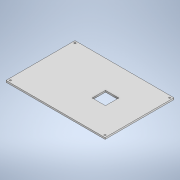
# Autodesk Inventor part: remoteswitchlid
Saved by Autodesk Inventor 2021 (Build 250183000, 183)
## iProperties
Created: 2021-10-23
Part Number: remoteswitchlid
Material: Generic
Document SubType Name: Modeling
Designer: eddys
Density: 1 g/cm^3
Appearance: Default
Author: eddys
Autodesk Inventor part; units mm, degrees
ref_plane "YZ Plane" through (0, 0, 0) normal (1, 0, 0) x (0, 1, 0)
ref_plane "XZ Plane" through (0, 0, 0) normal (0, 1, 0) x (-1, 0, 0)
ref_plane "XY Plane" through (0, 0, 0) normal (0, 0, 1) x (1, 0, 0)
sketch "Sketch1" plane through (0, 0, 0) normal (0, 1, 0) x (-1, 0, 0)
  line L0 (45.25, 31.5) -> (-45.25, 31.5)
  line L1 (-45.25, 31.5) -> (-45.25, -31.5)
  line L2 (-45.25, -31.5) -> (45.25, -31.5)
  line L3 (45.25, -31.5) -> (45.25, 31.5)
  line L4 (45.25, 31.5) -> (-45.25, -31.5) construction
  line L5 (-45.25, 31.5) -> (45.25, -31.5) construction
  point P0 (0, 0)
  dimension "d0" = 63
  dimension "d1" = 90.5
  constraints: 12 end point, 2 midpoint, 2 parallel, 1 horizontal, 1 perpendicular
  measures "d0" distance of L2.end L0.start
  measures "d1" distance of L1.end L2.end
extrude "Extrusion1" add sketch "Sketch1" along normal blind 1.5
sketch "Sketch2" plane through (0, 1.5, 0) normal (0, 1, 0) x (1, 0, 0)
  circle A0 centre (-43.25, -29.5) radius 0.75
  line L0 (-45.25, 31.5) -> (-45.25, -31.5) projected
  line L1 (-45.25, -31.5) -> (45.25, -31.5) projected
  circle A1 centre (-43.25, 29.5) radius 0.75
  line L2 (45.25, 31.5) -> (-45.25, 31.5) projected
  circle A2 centre (43.25, -29.5) radius 0.75
  line L3 (45.25, -31.5) -> (45.25, 31.5) projected
  circle A3 centre (43.25, 29.5) radius 0.75
  point P0 (0, 0)
  dimension "d4" = 2
  dimension "d5" = 2
  dimension "d6" = 1.5
  dimension "d7" = 2
  dimension "d8" = 2
  dimension "d9" = 1.5
  dimension "d10" = 2
  dimension "d11" = 2
  dimension "d12" = 1.5
  dimension "d13" = 1.5
  dimension "d14" = 2
  dimension "d15" = 2
  constraints: 4 centre point
  measures "d4" distance from line of L0 A0.centre
  measures "d5" distance from line of L1 A0.centre
  measures "d6" diameter of A0
  measures "d7" distance from line of L0 A1.centre
  measures "d8" distance from line of L2 A1.centre
  measures "d9" diameter of A1
  measures "d10" distance from line of L1 A2.centre
  measures "d11" distance from line of L3 A2.centre
  measures "d12" diameter of A2
  measures "d13" diameter of A3
  measures "d14" distance from line of L2 A3.centre
  measures "d15" distance from line of L3 A3.centre
extrude "Extrusion2" cut sketch "Sketch2" against normal blind 1.5 contours A0 | A1 | A2 | A3
sketch "Sketch6" plane through (0, 1.5, 0) normal (0, 1, 0) x (1, 0, 0)
  line L0 (8.05, -6.1) -> (20.25, -6.1)
  line L1 (20.25, -6.1) -> (20.25, 6.1)
  line L2 (20.25, 6.1) -> (8.05, 6.1)
  line L3 (8.05, 6.1) -> (8.05, -6.1)
  line L4 (-45.25, -31.5) -> (45.25, -31.5) projected
  line L5 (45.25, -31.5) -> (45.25, 31.5) projected
  point P0 (0, 0)
  dimension "d42" = 12.2
  dimension "d43" = 12.2
  dimension "d44" = 25.4
  dimension "d45" = 25
  constraints: 8 end point, 2 parallel, 1 horizontal, 1 perpendicular
  measures "d42" distance of L2.end L0.start
  measures "d43" distance of L0.start L0.end
  measures "d44" distance between parallel lines of L4 L0
  measures "d45" distance between parallel lines of L5 L1
extrude "Extrusion6" cut sketch "Sketch6" against normal blind 10
body "Solid1"
